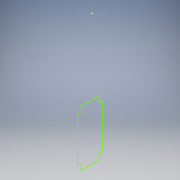
# Autodesk Inventor part: Part3
Saved by Autodesk Inventor 2016 (Build 200138000, 138)
## iProperties
Created: 2017-09-28
Part Number: Part3
Material: Generic
Document SubType Name: Modeling
Designer: student
Density: 1 g/cm^3
Appearance: Default
Author: student
Autodesk Inventor part; units mm, degrees
ref_plane "YZ Plane" through (0, 0, 0) normal (1, 0, 0) x (0, 1, 0)
ref_plane "XZ Plane" through (0, 0, 0) normal (0, 1, 0) x (-1, 0, 0)
ref_plane "XY Plane" through (0, 0, 0) normal (0, 0, 1) x (1, 0, 0)
sketch "Sketch1" plane through (0, 0, 0) normal (1, 0, 0) x (0, 1, 0)
  line L0 (-91.985, -4.7571) -> (-89.0815, -4.7571)
  line L1 (-89.0815, -4.7571) -> (-89.0815, -7.1749)
  line L2 (-89.0815, -7.1749) -> (-81.5711, -7.1749)
  line L3 (-57.4992, -7.1749) -> (-57.4992, -4.7571)
  line L4 (-57.4992, -4.7571) -> (-54.5957, -4.7571)
  line L5 (-54.5957, -4.7571) -> (-54.5957, -4.795)
  line L6 (-54.5957, -4.795) -> (-53.1756, -4.795)
  line L7 (-53.1756, -4.795) -> (-53.1756, 8.1844)
  line L8 (-53.1756, 8.1844) -> (-54.5957, 8.1844)
  line L9 (-54.5957, 8.1844) -> (-54.5957, 8.1465)
  line L10 (-54.5957, 8.1465) -> (-57.4992, 8.1465)
  line L11 (-57.4992, 8.1465) -> (-57.4992, 10.5643)
  line L12 (-57.4992, 10.5643) -> (-61.7845, 10.5643)
  line L13 (-89.0815, 10.5643) -> (-89.0815, 8.1465)
  line L14 (-89.0815, 8.1465) -> (-91.985, 8.1465)
  line L15 (-91.985, 8.1465) -> (-91.985, 8.1844)
  line L16 (-91.985, 8.1844) -> (-93.4052, 8.1844)
  line L17 (-93.4052, 8.1844) -> (-93.4052, -4.795)
  line L18 (-93.4052, -4.795) -> (-91.985, -4.795)
  line L19 (-91.985, -4.795) -> (-91.985, -4.7571)
  line L20 (-81.5711, 10.5643) -> (-89.0815, 10.5643)
  line L21 (-61.7845, -7.1749) -> (-57.4992, -7.1749)
  line L22 (-61.7845, 10.5643) -> (-81.5711, 10.5643)
  line L23 (-61.7845, -7.1749) -> (-81.5711, -7.1749)
  point P0 (0, 0)
  constraints: 48 end point, 1 horizontal, 1 parallel
extrude "Extrusion1" add sketch "Sketch1" along normal blind 2.921
body "Solid1"
